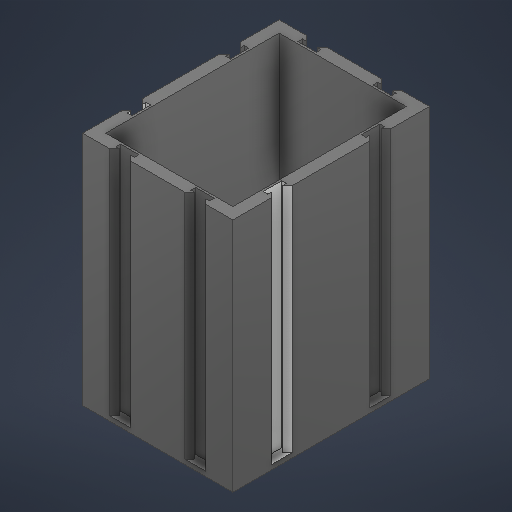
# Autodesk Inventor part: box
Saved by Autodesk Inventor 2027 (Build 310192060, 192F)
## iProperties
Created: 2026-06-08
Part Number: box
Material: Ogólny
Document SubType Name: Modeling
Designer: User
Density: 1 g/cm^3
Appearance: Domyślna
Author: User
Autodesk Inventor part; units mm, degrees
ref_plane "YZ Plane" through (0, 0, 0) normal (1, 0, 0) x (0, 1, 0)
ref_plane "XZ Plane" through (0, 0, 0) normal (0, 1, 0) x (-1, 0, 0)
ref_plane "XY Plane" through (0, 0, 0) normal (0, 0, 1) x (1, 0, 0)
sketch "Szkic1" plane through (0, 0, 0) normal (0, 1, 0) x (-1, 0, 0)
  line L0 (-32.5, -42.5) -> (32.5, -42.5)
  line L1 (32.5, -42.5) -> (32.5, 42.5)
  line L2 (32.5, 42.5) -> (-32.5, 42.5)
  line L3 (-32.5, 42.5) -> (-32.5, -42.5)
  line L4 (-32.5, -42.5) -> (32.5, 42.5) construction
  line L5 (32.5, -42.5) -> (-32.5, 42.5) construction
  line L6 (-27.5, -37.5) -> (27.5, -37.5)
  line L7 (27.5, -37.5) -> (27.5, 37.5)
  line L8 (27.5, 37.5) -> (-27.5, 37.5)
  line L9 (-27.5, 37.5) -> (-27.5, -37.5)
  line L10 (-27.5, -37.5) -> (27.5, 37.5) construction
  line L11 (27.5, -37.5) -> (-27.5, 37.5) construction
  line L12 (32.5, 42.5) -> (20.871, 42.5)
  line L13 (32.5, 42.5) -> (44.129, 42.5) construction
  line L14 (20.871, 42.5) -> (18.7497, 40.3787)
  line L15 (18.7497, 40.3787) -> (20.2497, 40.3787)
  line L16 (20.2497, 40.3787) -> (20.2497, 38.3787)
  line L17 (-32.5, 42.5) -> (-30.5, 42.5) construction
  line L18 (0, 37.5) -> (0, 42.5) construction
  line L19 (20.871, 42.5) -> (27.1515, 42.5) construction
  line L20 (11.6284, 42.5) -> (24.1515, 42.5) construction
  line L21 (20.2497, 38.3787) -> (16.2497, 38.3787)
  line L22 (16.2497, 38.3787) -> (16.2497, 42.5) construction
  line L23 (11.6284, 42.5) -> (13.7497, 40.3787)
  line L24 (13.7497, 40.3787) -> (12.2497, 40.3787)
  line L25 (12.2497, 40.3787) -> (12.2497, 38.3787)
  line L26 (12.2497, 38.3787) -> (16.2497, 38.3787)
  line L27 (-20.871, 42.5) -> (-18.7497, 40.3787)
  line L28 (-18.7497, 40.3787) -> (-20.2497, 40.3787)
  line L29 (-20.2497, 38.3787) -> (-16.2497, 38.3787)
  line L30 (-16.2497, 38.3787) -> (-16.2497, 42.5) construction
  line L31 (-11.6284, 42.5) -> (-13.7497, 40.3787)
  line L32 (-12.2497, 38.3787) -> (-16.2497, 38.3787)
  line L33 (-12.2497, 40.3787) -> (-12.2497, 38.3787)
  line L34 (-13.7497, 40.3787) -> (-12.2497, 40.3787)
  line L35 (-20.2497, 40.3787) -> (-20.2497, 38.3787)
  line L36 (27.5, 0) -> (-27.5, 0) construction
  line L37 (32.5, 42.5) -> (27.5, 37.5) construction
  line L38 (32.5, 0) -> (27.5, 0) construction
  line L39 (30.3787, -17.25) -> (28.3787, -17.25)
  line L40 (28.3787, -17.25) -> (28.3787, -21.25)
  line L41 (32.5, -16.6287) -> (30.3787, -18.75)
  line L42 (32.5, -25.8713) -> (30.3787, -23.75)
  line L43 (30.3787, -18.75) -> (30.3787, -17.25)
  line L44 (28.3787, -25.25) -> (28.3787, -21.25)
  line L45 (30.3787, -25.25) -> (28.3787, -25.25)
  line L46 (30.3787, -23.75) -> (30.3787, -25.25)
  line L47 (-28.3787, -25.25) -> (-28.3787, -21.25)
  line L48 (-28.3787, -17.25) -> (-28.3787, -21.25)
  line L49 (-30.3787, -25.25) -> (-28.3787, -25.25)
  line L50 (-30.3787, -23.75) -> (-30.3787, -25.25)
  line L51 (-32.5, -25.8713) -> (-30.3787, -23.75)
  line L52 (-30.3787, -17.25) -> (-28.3787, -17.25)
  line L53 (-30.3787, -18.75) -> (-30.3787, -17.25)
  line L54 (-32.5, -16.6287) -> (-30.3787, -18.75)
  line L55 (20.871, -42.5) -> (18.7497, -40.3787)
  line L56 (18.7497, -40.3787) -> (20.2497, -40.3787)
  line L57 (20.2497, -40.3787) -> (20.2497, -38.3787)
  line L58 (20.2497, -38.3787) -> (16.2497, -38.3787)
  line L59 (16.2497, -38.3787) -> (16.2497, -42.5) construction
  line L60 (11.6284, -42.5) -> (13.7497, -40.3787)
  line L61 (12.2497, -38.3787) -> (16.2497, -38.3787)
  line L62 (12.2497, -40.3787) -> (12.2497, -38.3787)
  line L63 (13.7497, -40.3787) -> (12.2497, -40.3787)
  line L64 (-11.6284, -42.5) -> (-13.7497, -40.3787)
  line L65 (-13.7497, -40.3787) -> (-12.2497, -40.3787)
  line L66 (-16.2497, -38.3787) -> (-16.2497, -42.5) construction
  line L67 (-12.2497, -38.3787) -> (-16.2497, -38.3787)
  line L68 (-20.871, -42.5) -> (-18.7497, -40.3787)
  line L69 (-18.7497, -40.3787) -> (-20.2497, -40.3787)
  line L70 (-20.2497, -38.3787) -> (-16.2497, -38.3787)
  line L71 (-12.2497, -40.3787) -> (-12.2497, -38.3787)
  line L72 (-20.2497, -40.3787) -> (-20.2497, -38.3787)
  line L73 (28.3787, -21.25) -> (32.5, -21.25) construction
  line L74 (28.3787, 25.25) -> (28.3787, 21.25)
  line L75 (28.3787, 17.25) -> (28.3787, 21.25)
  line L76 (30.3787, 25.25) -> (28.3787, 25.25)
  line L77 (30.3787, 23.75) -> (30.3787, 25.25)
  line L78 (32.5, 25.8713) -> (30.3787, 23.75)
  line L79 (30.3787, 17.25) -> (28.3787, 17.25)
  line L80 (30.3787, 18.75) -> (30.3787, 17.25)
  line L81 (32.5, 16.6287) -> (30.3787, 18.75)
  line L82 (-30.3787, 17.25) -> (-28.3787, 17.25)
  line L83 (-30.3787, 18.75) -> (-30.3787, 17.25)
  line L84 (-32.5, 16.6287) -> (-30.3787, 18.75)
  line L85 (-28.3787, 17.25) -> (-28.3787, 21.25)
  line L86 (-28.3787, 25.25) -> (-28.3787, 21.25)
  line L87 (-30.3787, 23.75) -> (-30.3787, 25.25)
  line L88 (-32.5, 25.8713) -> (-30.3787, 23.75)
  line L89 (-30.3787, 25.25) -> (-28.3787, 25.25)
  line L90 (28.3787, 21.25) -> (32.5, 21.25) construction
  point P0 (0, 0)
  point P1 (-11.6284, 42.5)
  point P2 (-20.871, 42.5)
  point P3 (-32.5, -16.6287)
  point P4 (-32.5, -25.8713)
  point P5 (-20.871, -42.5)
  point P6 (11.6284, -42.5)
  point P7 (20.871, -42.5)
  point P8 (32.5, -25.8713)
  point P9 (32.5, -16.6287)
  point P10 (20.871, 42.5)
  point P11 (17.8899, 42.5)
  point P12 (0, 40)
  point P13 (16.2497, 40.4393)
  point P14 (30, 0)
  point P15 (30.4393, -21.25)
  point P16 (30.4393, 21.25)
  dimension "d0" = 65
  dimension "d1" = 85
  dimension "d2" = 55
  dimension "d3" = 75
  dimension "d4" = 11.629
  dimension "d5" = 180
  dimension "d6" = 3
  dimension "d7" = 135
  dimension "d8" = 1.5
  dimension "d9" = 2
  dimension "d15" = 2
  dimension "d23" = 4
  dimension "d29" = 45
  dimension "d30" = 16.2497
  dimension "d31" = 21.25
  constraints: 182 end point, 62 symmetric about line, 14 midpoint, 6 point on line, 5 parallel, 5 perpendicular, 4 horizontal, 2 collinear, 2 vertical
  measures "d0" distance of L2.end L1.end
  measures "d1" distance of L1.end L0.end
  measures "d2" distance of L8.end L7.end
  measures "d3" distance of L7.end L6.end
  measures "d4" distance of L1.end L12.end
  measures "d5" angle of L12 L13
  measures "d6" distance of L12.end L14.end
  measures "d7" angle of L14 L12
  measures "d8" distance of L14.end L15.end
  measures "d9" distance of L15.end L16.end
  measures "d15" distance of L2.end L17.end
  measures "d23" distance of L16.end L21.end
  measures "d29" angle of L24 L23
  measures "d30" horizontal distance of point (0, 40) point (16.25, 40.439)
  measures "d31" vertical distance of point (30, 0) point (30.439, -21.25)
extrude "Wyciągnięcie proste1" add sketch "Szkic1" along normal blind 100 contours L3 L51 L50 L49 L47 L48 L52 L53 L54 L84 L83 L82 L85 L86 L89 L87 L88 L2 L27 L28 L35 L29 L32 L33 L34 L31 L23 L24 L25 L26 L21 L16 L15 L14 L1 L78 L77 L76 L74 L75 L79 L80 L81 L41 L43 L39 L40 L44 L45 L46 L42 L0 L55 L56 L57 L58 L61 L62 L63 L60 L64 L65 L71 L67 L70 L72 L69 L68
extrude "Wyciągnięcie proste2" add sketch "Szkic1" against normal blind 2 contours L3 L51 L50 L49 L47 L48 L52 L53 L54 L84 L83 L82 L85 L86 L89 L87 L88 L2 L27 L28 L35 L29 L32 L33 L34 L31 L23 L24 L25 L26 L21 L16 L15 L14 L1 L78 L77 L76 L74 L75 L79 L80 L81 L41 L43 L39 L40 L44 L45 L46 L42 L0 L55 L56 L57 L58 L61 L62 L63 L60 L64 L65 L71 L67 L70 L72 L69 L68 | L68 L69 L72 L70 L67 L71 L65 L64 L0 | L3 L54 L53 L52 L48 L47 L49 L50 L51 | L60 L63 L62 L61 L58 L57 L56 L55 L0 | L3 L88 L87 L89 L86 L85 L82 L83 L84 | L42 L46 L45 L44 L40 L39 L43 L41 L1 | L2 L31 L34 L33 L32 L29 L35 L28 L27 | L81 L80 L79 L75 L74 L76 L77 L78 L1 | L2 L14 L15 L16 L21 L26 L25 L24 L23 | L9 L8 L7 L6
